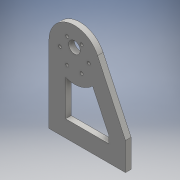
# Autodesk Inventor part: chassi_front_template
Saved by Autodesk Inventor 2016 (Build 200138000, 138)
## iProperties
Created: 2017-01-01
Part Number: chassi_front_template
Material: Generic
Document SubType Name: Modeling
Designer: hesaon
Density: 1 g/cm^3
Appearance: Default
Author: hesaon
Autodesk Inventor part; units mm, degrees
ref_plane "YZ Plane" through (0, 0, 0) normal (1, 0, 0) x (0, 1, 0)
ref_plane "XZ Plane" through (0, 0, 0) normal (0, 1, 0) x (-1, 0, 0)
ref_plane "XY Plane" through (0, 0, 0) normal (0, 0, 1) x (1, 0, 0)
sketch "Sketch1" plane through (0, 0, 0) normal (0, 1, 0) x (-1, 0, 0)
  line L0 (-55, -52.5) -> (-24.8972, 11.6781)
  line L1 (-55, -82.5) -> (-55, -52.5)
  line L2 (27.5, 0) -> (27.5, -82.5)
  line L3 (9.5, -64.5) -> (-37, -64.5)
  line L4 (9.5, -64.5) -> (9.5, -25.807)
  line L5 (-37, -64.5) -> (-37, -56.5118)
  arc A0 (27.5, 0) -> (-24.8972, 11.6781) centre (0, 0) ccw
  arc A1 (-19.56, -19.3302) -> (9.5, -25.807) centre (0, 0) ccw
  circle A2 centre (0, 7) radius 6.25
  circle A3 centre (15.5, 0) radius 1.6
  circle A4 centre (7.75, 13.4234) radius 1.6
  circle A5 centre (-7.75, 13.4234) radius 1.6
  circle A6 centre (-15.5, 0) radius 1.6
  circle A7 centre (-7.75, -13.4234) radius 1.6
  circle A8 centre (7.75, -13.4234) radius 1.6
  line L6 (-19.56, -19.3302) -> (-37, -56.5118)
  line L7 (27.5, -82.5) -> (-55, -82.5)
  dimension "d12" = 18
  dimension "d13" = 82.5
  dimension "d14" = 12.5
  dimension "d15" = 7
  dimension "d16" = 3.2
  dimension "d17" = 15.5
  dimension "d20" = 360
  dimension "d22" = 30
  dimension "d23" = 27.5
  dimension "d24" = 18
  dimension "d25" = 27.5
  dimension "d26" = 27.5
  dimension "d27" = 27.5
  dimension "d29" = 18
  dimension "d30" = 18
  dimension "d31" = 82.5
  dimension "d32" = 82.5
  constraints: 16 end point, 9 centre point, 4 point on circle, 3 vertical, 2 horizontal, 2 tangent, 1 horizontal alignment, 1 parallel, 1 vertical alignment, 13 other
  measures "d12" distance from line of L1 L3.end
  measures "d13" distance of L2.end L1.start
  measures "d14" diameter of A2
  measures "d15" distance of point (0, 0) A2.centre
  measures "d16" diameter of A3
  measures "d17" distance of point (0, 0) A3.centre
  measures "d22" distance of L1.start L0.start
  measures "d23" radius of A0
  measures "d24" distance between parallel lines of L4 L2
  measures "d25" radius of A1
  measures "d26" distance of L2.start point (0, 0)
  measures "d27" distance from line of L0 point (0, 0)
  measures "d29" distance between parallel lines of L0 L6
  measures "d30" distance between parallel lines of L7 L3
  measures "d31" distance from line of point (0, 0) L7
  measures "d32" distance of L2.end L2.start
extrude "Extrusion1" add sketch "Sketch1" along normal blind 6
body "Solid1"
